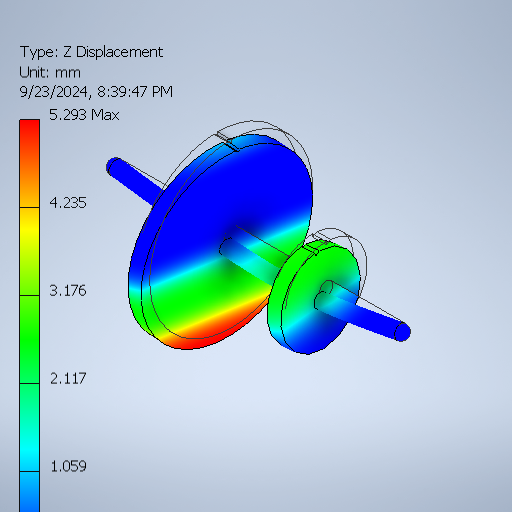
# Autodesk Inventor part: shaft_model
Saved by Autodesk Inventor 2025 (Build 290162000, 162)
## iProperties
Created: 2024-09-23
Part Number: shaft_model
Material: Steel
Document SubType Name: Modeling
Designer: brian_kob2vtf
Mass: 153817 g
Surface Area: 9984.2 cm^2
Volume: 19594.6 cm^3
Density: 7.85 g/cm^3
Appearance: Plate
Author: brian_kob2vtf
Autodesk Inventor part; units mm, degrees
ref_plane "YZ Plane" through (0, 0, 0) normal (1, 0, 0) x (0, 1, 0)
ref_plane "XZ Plane" through (0, 0, 0) normal (0, 1, 0) x (-1, 0, 0)
ref_plane "XY Plane" through (0, 0, 0) normal (0, 0, 1) x (1, 0, 0)
sketch "Sketch1" plane through (0, 0, 0) normal (0, 1, 0) x (-1, 0, 0)
  line L0 (0, 0) -> (-400, 0) construction
  line L1 (-400, 0) -> (-750, 0)
  line L2 (-750, 0) -> (-1050, 0)
  line L3 (-400, 0) -> (-400, -300) construction
  line L4 (-400, -300) -> (-375, -300) construction
  line L5 (-375, -300) -> (-425, -300)
  line L6 (-425, -300) -> (-425, 0)
  line L7 (-425, 0) -> (-375, 0)
  line L8 (-375, 0) -> (-375, -300)
  line L9 (0, 0) -> (-1050, 0)
  line L10 (-1050, 0) -> (-1050, -25)
  line L11 (-1050, -25) -> (0, -25)
  line L12 (0, -25) -> (0, 0)
  arc A0 (0, -25) -> (25, 0) centre (0, 0) ccw
  line L13 (0, 0) -> (25, 0) construction
  line L14 (-750, 0) -> (-750, -150) construction
  line L15 (-750, -150) -> (-725, -150) construction
  line L16 (-725, -150) -> (-775, -150)
  line L17 (-775, -150) -> (-775, 0)
  line L18 (-775, 0) -> (-725, 0)
  line L19 (-725, 0) -> (-725, -150)
  arc A1 (-1075, 0) -> (-1050, -25) centre (-1050, 0) ccw
  line L20 (-1050, 0) -> (-1075, 0)
  line L21 (25, 0) -> (0, 0)
  point P0 (-775, -25)
  point P1 (-725, -25)
  point P2 (-425, -25)
  point P3 (-375, -25)
  dimension "d0" = 400
  dimension "d1" = 350
  dimension "d2" = 300
  dimension "d3" = 300
  dimension "d4" = 25
  dimension "d5" = 50
  dimension "d6" = 1050
  dimension "d7" = 25
  dimension "d8" = 150
  dimension "d9" = 25
  dimension "d10" = 50
  constraints: 44 end point, 7 horizontal, 6 parallel, 6 perpendicular, 4 point on circle, 4 point on line, 2 centre point, 2 coincident, 1 tangent, 1 vertical
  measures "d0" distance of L0.start L0.end
  measures "d1" distance of L0.end L1.end
  measures "d2" distance of L1.end L2.end
  measures "d3" distance of L0.end L3.end
  measures "d4" distance of L3.end L4.end
  measures "d5" distance of L6.end L7.end
  measures "d6" distance of L10.end L11.end
  measures "d7" distance of L10.end L9.end
  measures "d8" distance of L1.end L14.end
  measures "d9" distance of L14.end L15.end
  measures "d10" distance of L17.end L18.end
revolve "Revolution1" add sketch "Sketch1" angle 360 about axis through (0, 0, 0) along (1, 0, 0)
sketch "Sketch2" plane through (375, 0, 0) normal (-1, 0, 0) x (0, 0, 1)
  circle A0 centre (0, 0) radius 300 projected
  line L0 (0, 300) -> (0, 290)
  line L1 (0, 290) -> (25.5833, 307.4702)
  point P0 (14.1547, 299.6659)
  dimension "d12" = 10
  constraints: 4 end point, 1 vertical, 2 other
  measures "d12" distance of L0.start L0.end
extrude "Extrusion1" cut sketch "Sketch2" against normal blind 284.25 contours A0 L1 L0 picked at (7.8644, 296.5058)
sketch "Sketch3" plane through (775, 0, 0) normal (1, 0, 0) x (0, 0, -1)
  circle A0 centre (0, 0) radius 150 projected
  line L0 (0, 150) -> (0, 140)
  line L1 (0, 140) -> (62.4254, 176.0413)
  point P0 (15.8635, 149.1588)
  dimension "d15" = 10
  dimension "d16" = 60
  constraints: 4 end point, 1 vertical, 2 other
  measures "d15" distance of L0.start L0.end
  measures "d16" angle of L1 L0
extrude "Extrusion2" cut sketch "Sketch3" against normal blind 139 contours A0 L1 L0 picked at (8.8167, 146.2616)
body "Solid1"
